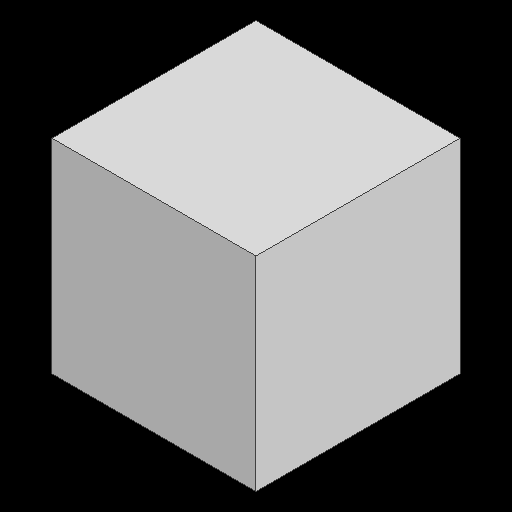
# Autodesk Inventor part: Part143
Saved by Autodesk Inventor 2025 (Build 290162000, 162)
## iProperties
Created: 2024-11-11
Part Number: Part143
Material: Generic
Document SubType Name: Modeling
Designer: Trevor
Density: 1 g/cm^3
Appearance: Default
Author: Trevor
Autodesk Inventor part; units mm, degrees
ref_plane "YZ Plane" through (0, 0, 0) normal (1, 0, 0) x (0, 1, 0)
ref_plane "XZ Plane" through (0, 0, 0) normal (0, 1, 0) x (-1, 0, 0)
ref_plane "XY Plane" through (0, 0, 0) normal (0, 0, 1) x (1, 0, 0)
sketch "Sketch1" plane through (0, 0, 0) normal (0, 1, 0) x (-1, 0, 0)
  line L0 (0, 0) -> (304.8, 0)
  line L1 (304.8, 0) -> (304.8, -304.8)
  line L2 (304.8, -304.8) -> (0, -304.8)
  line L3 (0, -304.8) -> (0, 0)
  dimension "d0" = 304.8
  dimension "d1" = 304.8
  constraints: 8 end point, 2 parallel, 1 horizontal, 1 perpendicular
  measures "d0" distance of L1.end L2.end
  measures "d1" distance of L0.end L1.end
extrude "Extrusion1" add sketch "Sketch1" along normal blind 304.8
ref_plane "Work Plane1" through (-304.8, 0, -304.8) normal (-1, 0, 0) x (0, 0, 1)
ref_plane "Work Plane2" through (0, 0, -304.8) normal (0, 0, -1) x (-1, 0, 0)
ref_plane "Work Plane3" through (-304.8, 0, 0) normal (0, 0, 1) x (1, 0, 0)
ref_plane "Work Plane4" through (0, 304.8, 0) normal (0, 1, 0) x (1, 0, 0)
ref_plane "Work Plane5" through (0, 0, 0) normal (1, 0, 0) x (0, 0, -1)
ref_plane "Work Plane6" through (0, 0, 0) normal (0, -1, 0) x (1, 0, 0)
sketch "Sketch2" plane through (0, 0, -304.8) normal (0, 0, -1) x (-1, 0, 0)
  line L0 (0, 0) -> (304.8, 0) construction
  line L1 (304.8, 0) -> (304.8, 304.8) construction
  line L2 (0, 304.8) -> (304.8, 304.8) construction
  line L3 (0, 0) -> (0, 304.8) construction
sketch "Sketch3" plane through (-304.8, 0, -304.8) normal (-1, 0, 0) x (0, 0, 1)
  line L0 (0, 0) -> (304.8, 0) construction
  line L1 (304.8, 0) -> (304.8, 304.8) construction
  line L2 (0, 304.8) -> (304.8, 304.8) construction
  line L3 (0, 0) -> (0, 304.8) construction
sketch "Sketch4" plane through (0, 304.8, 0) normal (0, 1, 0) x (1, 0, 0)
  line L0 (0, 304.8) -> (-304.8, 304.8) construction
  line L1 (-304.8, 304.8) -> (-304.8, 0) construction
  line L2 (-304.8, 0) -> (0, 0) construction
  line L3 (0, 0) -> (0, 304.8) construction
body "Solid1"
